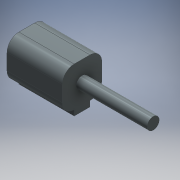
# Autodesk Inventor part: taladro
Saved by Autodesk Inventor 2016 (Build 200138000, 138)
## iProperties
Created: 2016-08-18
Part Number: taladro
Material: Iron, Ductile
Document SubType Name: Modeling
Designer: Admin
Density: 7.15 g/cm^3
Appearance: Iron Gray
Author: Admin
Autodesk Inventor part; units mm, degrees
ref_plane "YZ Plane" through (0, 0, 0) normal (1, 0, 0) x (0, 1, 0)
ref_plane "XZ Plane" through (0, 0, 0) normal (0, 1, 0) x (-1, 0, 0)
ref_plane "XY Plane" through (0, 0, 0) normal (0, 0, 1) x (1, 0, 0)
sketch "Sketch1" plane through (0, 0, 0) normal (1, 0, 0) x (0, 1, 0)
  line L0 (9.4737, 39.4737) -> (-40.5263, 39.4737)
  line L1 (-40.5263, 39.4737) -> (-40.5263, -10.5263)
  line L2 (-40.5263, -10.5263) -> (9.4737, -10.5263)
  line L3 (9.4737, -10.5263) -> (9.4737, 39.4737)
  point P0 (0, 0)
  dimension "d2" = 50
  dimension "d3" = 50
  constraints: 8 end point, 2 parallel, 1 horizontal, 1 perpendicular
  measures "d2" distance of L2.end L0.start
  measures "d3" distance of L1.end L2.end
extrude "Extrusion1" add sketch "Sketch1" along normal blind 70
sketch "Sketch2" plane through (70, 0, 0) normal (1, 0, 0) x (0, 0, -1)
  line L0 (-39.4737, 9.4737) -> (-39.4737, -40.5263) projected
  line L1 (-39.4737, -40.5263) -> (10.5263, -40.5263) projected
  line L2 (10.5263, 9.4737) -> (-39.4737, 9.4737) projected
  line L3 (10.5263, -40.5263) -> (10.5263, 9.4737) projected
  circle A0 centre (-14.4737, -15.5263) radius 7.5
  point P0 (0, 0)
  dimension "d7" = 15
  constraints: 1 centre point
  measures "d7" diameter of A0
extrude "Extrusion2" add sketch "Sketch2" along normal blind 90 contours A0
fillet "Fillet1" radius 15 4 edges at (35, 9.4737, 39.4737) (35, -40.5263, 39.4737) (35, 9.4737, -10.5263) (35, -40.5263, -10.5263)
sketch "Sketch3" plane through (0, -25.5263, -10.5263) normal (0, 0, -1) x (-1, 0, 0)
  line L0 (-70, 20) -> (-70, 35) projected
  line L1 (-70, 20) -> (0, 20)
  line L2 (0, 20) -> (0, 0)
  line L3 (0, 0) -> (-70, 0)
  line L4 (-70, 0) -> (-70, 20)
  point P0 (0, 25.5263)
  constraints: 8 end point, 2 parallel, 1 horizontal, 1 perpendicular
extrude "Extrusion3" add sketch "Sketch3" along normal blind 7
body "Solid1"
